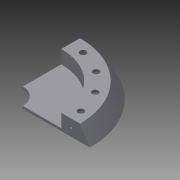
# Autodesk Inventor part: led
Saved by Autodesk Inventor 2014 (Build 180170000, 170)
## iProperties
Created: 2014-01-15
Part Number: led
Material: Générique
Document SubType Name: Modeling
Designer: helly
Density: 1 g/cm^3
Appearance: Par défaut
Author: helly
Autodesk Inventor part; units mm, degrees
ref_plane "YZ Plane" through (0, 0, 0) normal (1, 0, 0) x (0, 1, 0)
ref_plane "XZ Plane" through (0, 0, 0) normal (0, 1, 0) x (-1, 0, 0)
ref_plane "XY Plane" through (0, 0, 0) normal (0, 0, 1) x (1, 0, 0)
sketch "Esquisse4" plane through (0, 0, 0) normal (1, 0, 0) x (0, 1, 0)
  line L0 (0, 0) -> (80, 0) construction
  line L1 (0, 0) -> (0, 76) construction
  line L2 (0, 76) -> (32, 76) construction
  line L3 (32, 76) -> (80, 0) construction
  line L4 (67.3684, 0) -> (67.3684, 20) construction
  line L5 (67.3684, 20) -> (0, 20) construction
  line L6 (67.3684, 20) -> (59.3585, 32.6823)
  line L7 (0, 20) -> (0, 22)
  line L8 (59.3585, 32.6823) -> (44.3585, 32.6823)
  line L9 (44.3585, 32.6823) -> (44.3585, 20)
  line L10 (44.3585, 20) -> (46.3585, 20)
  line L11 (46.3585, 20) -> (46.3585, 32.6823) construction
  line L12 (46.3585, 32.6823) -> (46.3585, 30.6823) construction
  line L13 (46.3585, 30.6823) -> (60.6217, 30.6823) construction
  line L14 (46.3585, 30.6823) -> (46.3585, 20)
  line L15 (58.2562, 30.6823) -> (65.0029, 20)
  line L16 (60.6217, 30.6823) -> (58.9307, 29.6143) construction
  line L17 (46.3585, 30.6823) -> (58.2562, 30.6823)
  line L18 (65.0029, 20) -> (67.3684, 20)
  line L19 (0, 20) -> (44.3585, 20)
  line L20 (0, 22) -> (44.3585, 22)
  dimension "d23" = 80
  dimension "d24" = 76
  dimension "d25" = 32
  dimension "d27" = 20
  dimension "d28" = 15
  dimension "d29" = 2
  dimension "d30" = 15
  dimension "d31" = 2
  dimension "d32" = 2
  dimension "d33" = 2
  constraints: 42 end point, 14 point on line, 10 perpendicular, 3 collinear, 2 parallel, 1 horizontal
  measures "d23" distance of L0.start L0.end
  measures "d24" distance of L0.start L1.end
  measures "d25" distance of L1.end L2.end
  measures "d27" distance of L4.start L4.end
  measures "d28" distance of L4.end L6.end
  measures "d29" distance of L5.end L7.end
  measures "d30" distance of L6.end L8.end
  measures "d31" distance of L9.end L10.end
  measures "d32" distance of L11.end L12.end
  measures "d33" distance of L13.end L16.end
revolve "Révolution2" add sketch "Esquisse4" angle 90 about axis through (0, 0, 0) along (0, 0, -1)
sketch "Esquisse9" plane through (0, 0, 22) normal (0, 0, 1) x (-0.7071, 0.7071, 0)
  circle A0 centre (0, 0) radius 44.3585 projected
  circle A1 centre (0, 0) radius 13.5
  dimension "d35" = 27
  constraints: 1 centre point, 1 coincident
  measures "d35" diameter of A1
extrude "Extrusion3" cut sketch "Esquisse9" against normal blind 10 contours A1
sketch "Esquisse14" plane through (0, 44.3585, 32.6823) normal (-1, 0, 0) x (0, 0, 1)
  line L0 (0, 0) -> (-10.6823, 0) projected
  line L1 (-12.6823, 20.6444) -> (-12.6823, 23.0099) projected
  line L2 (-2, 13.8977) -> (-12.6823, 20.6444) projected
  line L3 (-2, 2) -> (-2, 13.8977) projected
  line L4 (-12.6823, -30.8585) -> (-12.6823, 2) projected
  line L5 (-12.6823, 20.6444) -> (-2, 13.8977)
  line L6 (-2, 13.8977) -> (-2, 0)
  line L7 (-2, 0) -> (-12.6823, 0)
  line L8 (-12.6823, 0) -> (-12.6823, 20.6444)
  point P0 (-32.6823, -44.3585)
  constraints: 8 end point, 4 point on line, 2 collinear
extrude "Extrusion8" add sketch "Esquisse14" against normal blind 2
sketch "Esquisse15" plane through (44.3585, 0, 32.6823) normal (0, -1, 0) x (1, 0, 0)
  line L0 (-30.8585, -10.6823) -> (-30.8585, -12.6823) projected
  line L1 (-30.8585, -12.6823) -> (2, -12.6823) projected
  line L2 (13.8977, -2) -> (20.6444, -12.6823) projected
  line L3 (0, 0) -> (0, -10.6823) projected
  line L4 (0, -10.6823) -> (-30.8585, -10.6823) projected
  line L5 (20.6444, -12.6823) -> (13.8977, -2)
  line L6 (13.8977, -2) -> (0, -2)
  line L7 (0, -2) -> (0, -12.6823)
  line L8 (0, -12.6823) -> (20.6444, -12.6823)
  point P0 (-44.3585, -32.6823)
  constraints: 8 end point, 3 perpendicular, 2 point on line, 1 collinear
extrude "Extrusion9" add sketch "Esquisse15" against normal blind 2
sketch "Esquisse17" plane through (44.3585, 0, 32.6823) normal (0, -1, 0) x (1, 0, 0)
  line L0 (-30.8585, -12.6823) -> (23.0099, -12.6823) projected
  line L1 (15, 0) -> (0, 0) projected
  line L2 (15, 0) -> (0, 0) construction
  line L3 (7.5, 0) -> (7.5, -12.6823) construction
  circle A0 centre (7.5, -6.3412) radius 1
  point P0 (-44.3585, -32.6823)
  dimension "d61" = 2
  constraints: 4 end point, 2 midpoint, 1 centre point, 1 collinear, 1 perpendicular, 1 point on line
  measures "d61" diameter of A0
extrude "Extrusion10" cut sketch "Esquisse17" against normal blind 2
sketch "Esquisse18" plane through (0, 44.3585, 32.6823) normal (-1, 0, 0) x (0, 0, 1)
  line L0 (-12.6823, -30.8585) -> (-12.6823, 23.0099) projected
  line L1 (0, 15) -> (0, 0) projected
  line L2 (0, 0) -> (0, 15) construction
  line L3 (0, 7.5) -> (-12.6823, 7.5) construction
  circle A0 centre (-6.3412, 7.5) radius 1
  point P0 (-32.6823, -44.3585)
  dimension "d64" = 2
  constraints: 4 end point, 2 midpoint, 1 centre point, 1 collinear, 1 perpendicular, 1 point on line
  measures "d64" diameter of A0
extrude "Extrusion11" cut sketch "Esquisse18" against normal blind 2
sketch "Esquisse19" plane through (0, 44.3585, 32.6823) normal (0, 0, 1) x (1, 0, 0)
  arc A0 (44.3585, -44.3585) -> (0, 0) centre (0, -44.3585) ccw projected
  line L0 (59.3585, -44.3585) -> (44.3585, -44.3585) projected
  arc A1 (59.3585, -44.3585) -> (0, 15) centre (0, -44.3585) ccw projected
  line L1 (0, -44.3585) -> (59.3585, -44.3585) construction
  line L2 (44.3585, -44.3585) -> (59.3585, -44.3585) construction
  line L3 (0, -44.3585) -> (50.0625, -12.4652) construction
  line L4 (37.4116, -20.5247) -> (50.0625, -12.4652) construction
  circle A2 centre (43.737, -16.495) radius 2.5
  circle A3 centre (29.7448, -1.8785) radius 2.5
  circle A4 centre (11.2242, 6.2707) radius 2.5
  circle A5 centre (-9.0051, 6.7122) radius 2.5
  circle A6 centre (-27.8636, -0.6215) radius 2.5
  circle A7 centre (-42.48, -14.6137) radius 2.5
  circle A8 centre (-50.6293, -33.1343) radius 2.5
  circle A9 centre (-51.0707, -53.3637) radius 2.5
  circle A10 centre (-43.737, -72.2221) radius 2.5
  circle A11 centre (-29.7448, -86.8385) radius 2.5
  circle A12 centre (-11.2242, -94.9878) radius 2.5
  circle A13 centre (9.0051, -95.4292) radius 2.5
  circle A14 centre (27.8636, -88.0956) radius 2.5
  circle A15 centre (42.48, -74.1034) radius 2.5
  circle A16 centre (50.6293, -55.5828) radius 2.5
  circle A17 centre (51.0707, -35.3534) radius 2.5
  dimension "d67" = 32.5
  dimension "d68" = 5
  dimension "d71" = 360
  constraints: 16 centre point, 8 end point, 3 collinear, 2 point on circle, 1 midpoint, 1 point on line, 33 other
  measures "d67" angle of L3 L1
  measures "d68" diameter of A2
extrude "Extrusion12" cut sketch "Esquisse19" against normal through all contours A2 | A3 | A4 | A17
